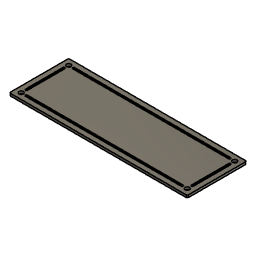
Flight Panel Blank (Autodesk Fusion 360 design; units mm, degrees)
Autodesk Fusion 360 part; units mm, degrees
other "Base Mesh Feature2"
mesh_to_body "Convert Mesh1" makes body 1
sketch "Sketch1" plane through (0, 0, 0) normal (0, 1, 0) x (1, 0, 0)
  line L0 (-90, 30) -> (90, 30)
  line L1 (90, 30) -> (90, -30)
  line L2 (90, -30) -> (-90, -30)
  line L3 (-90, -30) -> (-90, 30)
  line L4 (0, 30) -> (0, -30) construction
  dimension "d2" = 180
  dimension "d3" = 60
  constraint horizontal L0
  constraint vertical L1
  constraint horizontal L2
  constraint vertical L3
  constraint midpoint L0 L4.start
  constraint midpoint L2 L4.end
  constraint midpoint origin L4
  measures "d2" distance of L0.start L0.end
  measures "d3" distance of L0.start L2.end
extrude "Extrude1" add sketch "Sketch1" along normal blind 2.4 separate body makes body 2
other "Modify3"
move_body "Move1" [suppressed]
fillet "Fillet1" radius 1 4 edges at (90, 1.2, 30) (90, 1.2, -30) (-90, 1.2, -30) (-90, 1.2, 30) on bodies 2
sketch "Sketch2" plane through (0, 2.4, 0) normal (0, 1, 0) x (-1, 0, 0)
  arc A0 (90, 29) -> (89, 30) centre (89, 29) ccw
  line L0 (89, 30) -> (-89, 30)
  arc A1 (-89, 30) -> (-90, 29) centre (-89, 29) ccw
  line L1 (-90, 29) -> (-90, -29)
  arc A2 (-90, -29) -> (-89, -30) centre (-89, -29) ccw
  line L2 (-89, -30) -> (89, -30)
  arc A3 (89, -30) -> (90, -29) centre (89, -29) ccw
  line L3 (90, -29) -> (90, 29)
  line L4 (-79, -23) -> (79, -23)
  line L5 (79, -23) -> (79, -25)
  line L6 (79, -25) -> (-79, -25)
  line L7 (-79, -25) -> (-79, -23)
  line L8 (0, -30) -> (0, -25) construction
  dimension "d13" = 158
  dimension "d14" = 2
  dimension "d15" = 5
  constraint horizontal L4
  constraint vertical L5
  constraint horizontal L6
  constraint vertical L7
  constraint midpoint L2 L8.start
  constraint midpoint L6 L8.end
  measures "d13" distance of L5.end L6.end
  measures "d14" distance of L4.end L5.end
  measures "d15" distance of L8.start L8.end
extrude "Extrude2" add sketch "Sketch2" along normal blind 0.6 contours L4 L5 L6 L7 bodies 2
chamfer "Chamfer1" distance 0.6 angle 45 2 edges at (0, 3, -25) (0, 3, -23) on bodies 2
sketch "Sketch3" plane through (79, 0, 0) normal (1, 0, 0) x (0, 0, -1)
  line L0 (23.6, 3) -> (23, 2.4)
  line L1 (23, 2.4) -> (25, 2.4)
  line L2 (25, 2.4) -> (24.4, 3)
  line L3 (24.4, 3) -> (23.6, 3)
  line L4 (24, 3) -> (24, 2.4)
  line L5 (24, 3) -> (24.4, 3)
  line L6 (24.4, 3) -> (25, 2.4)
  line L7 (25, 2.4) -> (24, 2.4)
  constraint midpoint L3 L4.start
  constraint midpoint L1 L4.end
  constraint coincident L2.end L3.start
  constraint coincident L1.end L2.start
revolve "Revolve1" add sketch "Sketch3" angle 180 about axis through (79, 3, -24) along (0, -1, 0) contours L1 L2 L3 L4 L5 L6 L7 bodies 2
sketch "Sketch4" plane through (-79, 0, 0) normal (-1, 0, 0) x (0, 0, 1)
  line L0 (-23, 2.4) -> (-23.6, 3)
  line L1 (-23.6, 3) -> (-24.4, 3)
  line L2 (-24.4, 3) -> (-25, 2.4)
  line L3 (-25, 2.4) -> (-23, 2.4)
  line L4 (-24, 3) -> (-24, 2.4)
  line L5 (-24, 3) -> (-23.6, 3)
  line L6 (-23.6, 3) -> (-23, 2.4)
  constraint midpoint L1 L4.start
  constraint midpoint L3 L4.end
  constraint coincident L0.end L1.start
  constraint coincident L0.start L3.end
revolve "Revolve2" add sketch "Sketch4" angle 180 about axis through (-79, 3, -24) along (0, -1, 0) contours L0 L1 L3 L4 L5 L6 bodies 2
mirror "Mirror1" about plane through (0, 0, 0) normal (0, 0, 1) of "Extrude2", "Chamfer1", "Revolve1", "Revolve2"
sketch "Sketch5" plane through (0, 2.4, 0) normal (0, 1, 0) x (-1, 0, 0)
  arc A0 (79, 23) -> (79, 25) centre (79, 24) ccw
  line L0 (79, 23) -> (-79, 23)
  arc A1 (-79, 25) -> (-79, 23) centre (-79, 24) ccw
  line L1 (-79, 25) -> (79, 25)
  arc A2 (79, -25) -> (79, -23) centre (79, -24) ccw
  line L2 (79, -25) -> (-79, -25)
  arc A3 (-79, -23) -> (-79, -25) centre (-79, -24) ccw
  line L3 (-79, -23) -> (79, -23)
  arc A4 (90, 29) -> (89, 30) centre (89, 29) ccw
  line L4 (89, 30) -> (-89, 30)
  arc A5 (-89, 30) -> (-90, 29) centre (-89, 29) ccw
  line L5 (-90, 29) -> (-90, -29)
  arc A6 (-90, -29) -> (-89, -30) centre (-89, -29) ccw
  line L6 (-89, -30) -> (89, -30)
  arc A7 (89, -30) -> (90, -29) centre (89, -29) ccw
  line L7 (90, -29) -> (90, 29)
  line L8 (85, -19) -> (83, -19)
  line L9 (83, -19) -> (83, 19)
  line L10 (83, 19) -> (85, 19)
  line L11 (85, 19) -> (85, -19)
  line L12 (90, 0) -> (85, 0) construction
  dimension "d18" = 38
  dimension "d19" = 2
  dimension "d20" = 5
  constraint horizontal L8
  constraint vertical L9
  constraint horizontal L10
  constraint vertical L11
  constraint midpoint L7 L12.start
  constraint midpoint L11 L12.end
  constraint horizontal L12
  measures "d18" distance of L8.start L10.end
  measures "d19" distance of L8.start L8.end
  measures "d20" distance of L12.start L12.end
extrude "Extrude3" add sketch "Sketch5" along normal blind 0.6 contours L8 L9 L10 L11 bodies 2
chamfer "Chamfer2" distance 0.6 angle 45 2 edges at (-83, 3, 0) (-85, 3, 0) on bodies 2
sketch "Sketch6" plane through (0, 0, 19) normal (0, 0, 1) x (1, 0, 0)
  line L0 (-84.4, 3) -> (-85, 2.4)
  line L1 (-85, 2.4) -> (-83, 2.4)
  line L2 (-83, 2.4) -> (-83.6, 3)
  line L3 (-83.6, 3) -> (-84.4, 3)
  line L4 (-84, 3) -> (-84, 2.4)
  line L5 (-84, 3) -> (-83.6, 3)
  line L6 (-83.6, 3) -> (-83, 2.4)
  line L7 (-83, 2.4) -> (-84, 2.4)
  constraint midpoint L3 L4.start
  constraint midpoint L1 L4.end
  constraint coincident L2.end L3.start
  constraint coincident L1.end L2.start
revolve "Revolve3" add sketch "Sketch6" angle 180 about axis through (-84, 3, 19) along (0, -1, 0) contours L1 L2 L3 L4 L5 L6 L7 bodies 2
sketch "Sketch7" plane through (0, 0, -19) normal (0, 0, -1) x (-1, 0, 0)
  line L0 (85, 2.4) -> (84.4, 3)
  line L1 (84.4, 3) -> (83.6, 3)
  line L2 (83.6, 3) -> (83, 2.4)
  line L3 (83, 2.4) -> (85, 2.4)
  line L4 (84, 3) -> (84, 2.4)
  line L5 (84, 3) -> (84.4, 3)
  line L6 (84.4, 3) -> (85, 2.4)
  line L7 (85, 2.4) -> (84, 2.4)
  constraint midpoint L1 L4.start
  constraint midpoint L3 L4.end
  constraint coincident L0.end L1.start
  constraint coincident L0.start L3.end
revolve "Revolve4" add sketch "Sketch7" angle 180 about axis through (-84, 3, -19) along (0, -1, 0) contours L0 L1 L3 L4 L5 L6 L7 bodies 2
mirror "Mirror2" about plane through (0, 0, 0) normal (1, 0, 0) of "Extrude3", "Chamfer2", "Revolve3", "Revolve4"
sketch "Sketch8" plane through (0, 2.4, 0) normal (0, 1, 0) x (-1, 0, 0)
  arc A0 (-85, -19) -> (-83, -19) centre (-84, -19) ccw
  line L0 (-85, -19) -> (-85, 19)
  arc A1 (-83, 19) -> (-85, 19) centre (-84, 19) ccw
  line L1 (-83, 19) -> (-83, -19)
  arc A2 (83, -19) -> (85, -19) centre (84, -19) ccw
  line L2 (83, -19) -> (83, 19)
  arc A3 (85, 19) -> (83, 19) centre (84, 19) ccw
  line L3 (85, 19) -> (85, -19)
  arc A4 (79, 23) -> (79, 25) centre (79, 24) ccw
  line L4 (79, 23) -> (-79, 23)
  arc A5 (-79, 25) -> (-79, 23) centre (-79, 24) ccw
  line L5 (-79, 25) -> (79, 25)
  arc A6 (79, -25) -> (79, -23) centre (79, -24) ccw
  line L6 (79, -25) -> (-79, -25)
  arc A7 (-79, -23) -> (-79, -25) centre (-79, -24) ccw
  line L7 (-79, -23) -> (79, -23)
  arc A8 (90, 29) -> (89, 30) centre (89, 29) ccw
  line L8 (89, 30) -> (-89, 30)
  arc A9 (-89, 30) -> (-90, 29) centre (-89, 29) ccw
  line L9 (-90, 29) -> (-90, -29)
  arc A10 (-90, -29) -> (-89, -30) centre (-89, -29) ccw
  line L10 (-89, -30) -> (89, -30)
  arc A11 (89, -30) -> (90, -29) centre (89, -29) ccw
  line L11 (90, -29) -> (90, 29)
  circle A12 centre (-84, 24) radius 2.25
  dimension "d28" = 4.5
  dimension "d29" = 6
  dimension "d30" = 6
  measures "d28" diameter of A12
  measures "d29" distance of L8 A12.centre
  measures "d30" distance of L9 A12.centre
extrude "Extrude4" cut sketch "Sketch8" against normal up to surface (2.4 mm away) contours A12 bodies 2
mirror "Mirror3" about plane through (0, 0, 0) normal (0, 0, 1) of "Extrude4"
mirror "Mirror4" about plane through (0, 0, 0) normal (1, 0, 0) of "Extrude4", "Mirror3"
named bodies: "PNL-Mags-Lights-Fuel-Xtra"
